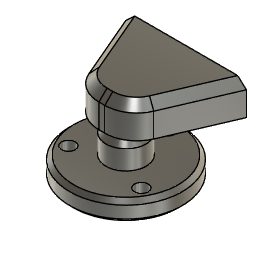
Omniwheel Caster v4 (Autodesk Fusion 360 design; units mm, degrees)
Autodesk Fusion 360 part; units mm, degrees
sketch "Sketch1" plane through (0, 0, 0) normal (0, 0, 1) x (1, 0, 0)
  circle A0 centre (0, 0) radius 14
  circle A1 centre (0, 0) radius 1.65
  circle A2 centre (0, 0) radius 10.5 construction
  circle A3 centre (0, 10.5) radius 1.7
  line L0 (0, 10.5) -> (0, 0) construction
  circle A4 centre (-9.0933, -5.25) radius 1.7
  circle A5 centre (9.0933, -5.25) radius 1.7
  dimension "d1" = 28
  dimension "d2" = 3.3
  dimension "d3" = 21
  dimension "d4" = 3.4
  dimension "d6" = 360
  constraint coincident A0.centre A1.centre
  constraint concentric A0 A1
  constraint concentric A0 A2
  constraint coincident A2 A3.centre
  constraint coincident A3.centre L0.start
  constraint vertical L0
  measures "d1" diameter of A0
  measures "d2" diameter of A1
  measures "d3" diameter of A2
  measures "d4" diameter of A3
extrude "Extrude1" add sketch "Sketch1" along normal blind 5 makes body 1
chamfer "Chamfer1" distance 1 angle 45 2 edges at (-13.0526, -5.0626, 5) (-13.0526, -5.0626, 0) on bodies 1
extrude "Extrude2" add sketch "Sketch1" along normal blind 4.5 contours A1 bodies 1
sketch "Sketch3" plane through (0, 0, 5) normal (0, 0, 1) x (-1, 0, 0)
  circle A0 centre (9.0933, 5.25) radius 1.7
  circle A1 centre (0, -10.5) radius 1.7
  circle A2 centre (-9.0933, 5.25) radius 1.7
  circle A3 centre (0, 0) radius 1.65
  circle A4 centre (0, 0) radius 13
  circle A5 centre (0, 0) radius 5
  dimension "d13" = 10
  constraint concentric A3 A5
  measures "d13" diameter of A5
extrude "Extrude3" add sketch "Sketch3" along normal blind 13 from surface at -5 contours A5 bodies 1
chamfer "Chamfer3" distance 3.2 angle 45 1 edges at (4.6616, 1.8081, 13) on bodies 1
sketch "Sketch4" plane through (0, 0, 13) normal (0, 0, 1) x (-1, 0, 0)
  circle A0 centre (0, 0) radius 1.65
  circle A1 centre (0, 0) radius 1.8
  line L0 (6, 6) -> (-6, 6)
  line L1 (-6, 6) -> (-6, -6)
  line L2 (-6, -6) -> (6, -6)
  line L3 (6, -6) -> (6, 6)
  line L4 (6, 6) -> (-6, -6) construction
  line L5 (-6, 6) -> (6, -6) construction
  line L6 (0, 0) -> (0, -15) construction
  line L7 (15, -15) -> (-15, -15)
  line L8 (15, -15) -> (6, 6)
  line L9 (-6, 6) -> (-15, -15)
  dimension "d18" = 12
  dimension "d19" = 12
  dimension "d23" = 15
  dimension "d24" = 30
  constraint horizontal L0
  constraint perpendicular L0 L1
  constraint parallel L0 L2
  constraint parallel L1 L3
  constraint coincident L4 A0.centre
  constraint coincident L5 A0.centre
  constraint coincident A0.centre A1.centre
  constraint vertical L6
  constraint perpendicular L6 L7
  constraint midpoint L6.end L7
  measures "d18" distance of L1.end L2.end
  measures "d19" distance of L0.end L1.end
  measures "d23" distance of A0.centre L6.end
  measures "d24" distance of L7.start L7.end
extrude "Extrude4" add sketch "Sketch4" along normal blind 8 separate body contours A0 | A1 | L0 L1 L2 L3 | L1 L2 L3 L7 L8 L9 makes body 2
fillet "Fillet1" radius 8 2 edges at (-6, -6, 17) (6, -6, 17) on bodies 2
extrude "Extrude5" cut sketch "Sketch4" along normal blind 3.7 contours A0 bodies 2
sketch "Sketch5" plane through (0, 15, 0) normal (0, 1, 0) x (-1, 0, 0)
  line L0 (-15, 21) -> (-15, 13)
  line L1 (-15, 13) -> (15, 13)
  line L2 (15, 13) -> (15, 21)
  line L3 (15, 21) -> (-15, 21)
  circle A0 centre (-11, 17) radius 1.5
  line L4 (0, 20) -> (0, 2.5)
  circle A1 centre (11, 17) radius 1.5
  dimension "d33" = 3
  dimension "d36" = 4
  dimension "d37" = 4
  constraint symmetric A0 L4 A1
  measures "d33" diameter of A0
  measures "d36" distance of L3 A0.centre
  measures "d37" distance of L0 A0.centre
extrude "Extrude6" cut sketch "Sketch5" against normal blind 5 contours A0 | A1 bodies 2
chamfer "Chamfer4" distance 2 angle 45 3 edges at (11.539, 6.9243, 21) (-11.539, 6.9243, 21) (5.1288, -4.6787, 21) on bodies 2
